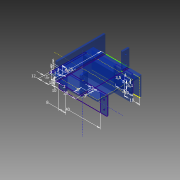
# Autodesk Inventor part: Joint
Saved by Autodesk Inventor 2015 (Build 190159000, 159)
## iProperties
Created: 2015-10-10
Part Number: Joint
Material: Generic
Document SubType Name: Modeling
Designer: styku
Density: 1 g/cm^3
Appearance: Clear - Blue
Mass: 14.9198 g
Surface Area: 152.062 cm^2
Volume: 14.9198 cm^3
Author: styku
Autodesk Inventor part; units mm, degrees
ref_plane "YZ Plane" through (0, 0, 0) normal (1, 0, 0) x (0, 1, 0)
ref_plane "XZ Plane" through (0, 0, 0) normal (0, 1, 0) x (-1, 0, 0)
ref_plane "XY Plane" through (0, 0, 0) normal (0, 0, 1) x (1, 0, 0)
sketch "Sketch1" plane through (0, 0, 0) normal (0, 1, 0) x (-1, 0, 0)
  line L0 (31, 0) -> (-47, 0) construction
  line L1 (0, 43) -> (0, -45) construction
  line L2 (20, 10) -> (-20, 10)
  line L3 (-20, 10) -> (-20, -10)
  line L4 (20, -10) -> (20, 10)
  line L5 (28, 12) -> (-28, 12)
  line L6 (-28, 12) -> (-28, -10)
  line L7 (28, -10) -> (28, 12)
  circle A0 centre (24.25, 5) radius 0.5
  line L8 (-20, -10) -> (-28, -10)
  line L9 (20, -10) -> (28, -10)
  circle A1 centre (24.25, -5) radius 0.5
  circle A2 centre (-24.25, 5) radius 0.5
  circle A3 centre (-24.25, -5) radius 0.5
  line L10 (-20, 10) -> (-28, 10)
  line L11 (20, 10) -> (28, 10)
  line L12 (-20, -10) -> (20, -10)
  point P0 (0, 0)
  dimension "d1" = 40
  dimension "d3" = 8
  dimension "d4" = 1
  dimension "d5" = 4.25
  dimension "d6" = 5
  dimension "d7" = 2
  dimension "d8" = 10
  dimension "d9" = 10
  constraints: 26 end point, 4 centre point, 4 horizontal, 3 parallel, 3 perpendicular, 3 point on line, 3 symmetric about line, 2 vertical, 1 collinear, 5 other
  measures "d1" distance between parallel lines of L3 L4
  measures "d3" distance between parallel lines of L4 L7
  measures "d4" diameter of A0
  measures "d5" distance from line of L4 A0.centre
  measures "d6" distance from line of L2 A0.centre
  measures "d7" distance between parallel lines of L2 L5
  measures "d8" distance between parallel lines of L0 L2
  measures "d9" distance between parallel lines of L9 L0
extrude "Extrusion1" add sketch "Sketch1" along normal blind 2 contours L11 L7 L9 L4 | L2 L10 L6 L5 L7 L11 | L3 L8 L6 L10
extrude "Extrusion2" add sketch "Sketch1" along normal blind 30 contours L2 L10 L6 L5 L7 L11
extrude "Extrusion3" add sketch "Sketch1" against normal blind 11 contours L2 L10 L6 L5 L7 L11
sketch "Sketch2" plane through (28, 0, 10) normal (0, 0, -1) x (-1, 0, 0)
  line L0 (0, 30) -> (56, 30) projected
  line L1 (56, 30) -> (56, 28)
  line L2 (56, -11) -> (56, 30) projected
  line L3 (56, 28) -> (0, 28)
  line L4 (0, 28) -> (0, 30)
  line L5 (0, 2) -> (0, 30) projected
  point P0 (28, 0)
  dimension "d18" = 2
  constraints: 6 end point, 1 collinear, 1 perpendicular, 1 point on line
  measures "d18" distance of L0.end L1.end
extrude "Extrusion4" add sketch "Sketch2" along normal blind 20
sketch "Sketch4" plane through (-28, 30, 12) normal (0, 0, 1) x (1, 0, 0)
  line L0 (56, -41) -> (0, -41) construction
  line L1 (0, -41) -> (0, 0) construction
  line L2 (0, 0) -> (56, 0) construction
  line L3 (56, -41) -> (56, 0) construction
  line L4 (12, -46) -> (12, 10)
  line L5 (12, 10) -> (14, 10)
  line L6 (14, 10) -> (14, -46)
  line L7 (14, -46) -> (12, -46)
  line L8 (42, -46) -> (40, -46)
  line L9 (40, -46) -> (40, -38)
  line L10 (40, -38) -> (42, -38)
  line L11 (42, -38) -> (42, -46)
  line L12 (66, -18) -> (-18, -18) construction
  line L13 (42, 10) -> (40, 10)
  line L14 (40, 10) -> (40, 2)
  line L15 (40, 2) -> (42, 2)
  line L16 (42, 2) -> (42, 10)
  line L17 (42, -46) -> (12, -46)
  line L18 (12, -46) -> (12, 10)
  line L19 (12, 10) -> (42, 10)
  line L20 (42, 10) -> (42, -46)
  line L21 (0, 0) -> (2, 0)
  line L22 (2, 0) -> (2, -41)
  line L23 (2, -41) -> (0, -41)
  line L24 (0, -41) -> (0, 0)
  point P0 (28, -30)
  dimension "d32" = 2
  dimension "d33" = 12
  dimension "d35" = 56
  dimension "d36" = 2
  dimension "d37" = 8
  dimension "d38" = 3
  dimension "d39" = 28
  dimension "d52" = 2
  constraints: 42 end point, 6 parallel, 4 horizontal, 4 perpendicular, 4 symmetric about line, 1 collinear, 1 point on line, 1 vertical
  measures "d32" distance between parallel lines of L6 L4
  measures "d33" distance between parallel lines of L1 L4
  measures "d35" distance between parallel lines of L7 L5
  measures "d36" distance of L9.end L10.end
  measures "d37" distance of L8.end L9.end
  measures "d38" distance between parallel lines of L0 L10
  measures "d39" distance between parallel lines of L6 L11
  measures "d52" distance between parallel lines of L1 L22
extrude "Extrusion7" add sketch "Sketch4" along normal blind 20 contours L4 L5 L6 L7 | L9 L10 L11 L8 | L13 L16 L15 L14
extrude "Extrusion8" add sketch "Sketch4" against normal blind 2 contours L4 L5 L6 L7 | L6 L19 L14 L15 L20 L10 L9 L17 | L9 L10 L11 L8 | L13 L16 L15 L14
sketch "Sketch5" plane through (14, -11, 12) normal (1, 0, 0) x (0, 0, -1)
  line L0 (-20, -5) -> (-20, 3) construction
  line L1 (2, -5) -> (-20, -5) construction
  line L2 (-20, 3) -> (-20, 51) construction
  line L3 (-20, 51) -> (-20, 51) construction
  line L4 (-20, 51) -> (2, 51) construction
  circle A0 centre (-15, -1.25) radius 0.5
  line L5 (0, 3) -> (-20, 3) construction
  line L6 (0, -5) -> (0, 3) construction
  line L7 (-10, -8) -> (-10, 8) construction
  line L8 (8, 23) -> (-29, 23) construction
  circle A1 centre (-5, -1.25) radius 0.5
  circle A2 centre (-15, 47.25) radius 0.5
  circle A3 centre (-5, 47.25) radius 0.5
  point P0 (12, 11)
  dimension "d44" = 1
  dimension "d45" = 5
  dimension "d46" = 4.25
  dimension "d47" = 10
  dimension "d49" = 20
  constraints: 4 centre point, 4 end point, 3 symmetric about line, 1 horizontal, 1 vertical, 3 other
  measures "d44" diameter of A0
  measures "d45" distance from line of L0 A0.centre
  measures "d46" distance from line of L5 A0.centre
  measures "d47" distance between parallel lines of L0 L7
  measures "d49" distance between parallel lines of L8 L5
extrude "Extrusion9" cut sketch "Sketch5" against normal blind 6
sketch "Sketch6" plane through (0, 30, 0) normal (0, 1, 0) x (1, 0, 0)
  line L0 (28, -12) -> (-28, -12)
  line L1 (-28, -12) -> (-28, -10)
  line L2 (-28, -10) -> (28, -10)
  line L3 (28, -10) -> (28, -12)
  point P0 (0, 0)
  constraints: 8 end point, 2 parallel, 1 horizontal, 1 perpendicular
extrude "Extrusion11" add sketch "Sketch6" along normal blind 10
sketch "Sketch7" plane through (-28, 30, 10) normal (0, 0, -1) x (-1, 0, 0)
  line L0 (0, 0) -> (0, 10) projected
  line L1 (-56, 10) -> (0, 10)
  line L2 (0, 10) -> (0, 8)
  line L3 (0, 8) -> (-56, 8)
  line L4 (-56, 8) -> (-56, 10)
  point P0 (-28, -30)
  dimension "d57" = 2
  constraints: 8 end point, 2 parallel, 1 horizontal, 1 perpendicular, 1 point on line
  measures "d57" distance between parallel lines of L3 L1
extrude "Extrusion12" add sketch "Sketch7" along normal blind 20
sketch "Sketch9" plane through (-28, 38, 10) normal (0, -1, 0) x (1, 0, 0)
  line L0 (56, 0) -> (56, -20) construction
  circle A0 centre (38, -10) radius 1.75
  line L1 (56, -20) -> (0, -20) construction
  line L2 (38, -13.05) -> (35.3586, -11.525)
  line L3 (35.3586, -11.525) -> (35.3586, -8.475)
  line L4 (35.3586, -8.475) -> (38, -6.95)
  line L5 (38, -6.95) -> (40.6414, -8.475)
  line L6 (40.6414, -8.475) -> (40.6414, -11.525)
  line L7 (40.6414, -11.525) -> (38, -13.05)
  line L8 (42, 0) -> (56, 0) projected
  line L9 (56, -20) -> (0, -20) projected
  line L10 (48, 0) -> (28, 0)
  line L11 (28, 0) -> (28, -20)
  line L12 (28, -20) -> (48, -20)
  line L13 (48, -20) -> (48, 0)
  line L14 (50, -10) -> (29, -10) construction
  line L15 (38, -1.4358) -> (38, -18.5642) construction
  point P0 (28, -10)
  dimension "d63" = 3.5
  dimension "d64" = 18
  dimension "d65" = 10
  dimension "d66" = 6.1
  dimension "d67" = 20
  constraints: 24 end point, 3 parallel, 2 horizontal, 2 midpoint, 2 perpendicular, 2 point on line, 1 centre point, 1 coincident, 1 vertical, 14 other
  measures "d63" diameter of A0
  measures "d64" distance from line of L0 A0.centre
  measures "d65" distance from line of L1 A0.centre
  measures "d66" distance of L2.start L4.end
  measures "d67" distance of L12.end L11.end
extrude "Extrusion13" add sketch "Sketch9" along normal blind 2.5 contours L8 L13 L9 L11 L10
extrude "Extrusion14" cut sketch "Sketch9" against normal blind 7.5 contours A0
body "Solid1"
